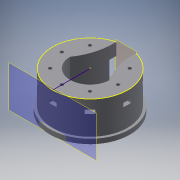
# Autodesk Inventor part: rotacion2_top
Saved by Autodesk Inventor 2017 (Build 210142000, 142)
## iProperties
Created: 2016-09-28
Part Number: rotacion2_top
Material: Generic
Document SubType Name: Modeling
Designer: Bardo91
Density: 1 g/cm^3
Appearance: Default
Author: Bardo91
Autodesk Inventor part; units mm, degrees
ref_plane "YZ Plane" through (0, 0, 0) normal (1, 0, 0) x (0, 1, 0)
ref_plane "XY Plane" through (0, 0, 0) normal (0, 0, 1) x (1, 0, 0)
sketch "Sketch1" plane through (0, 0, 0) normal (0, 0, 1) x (1, 0, 0)
  line L0 (0, -11) -> (-10.5, -11)
  line L1 (-10.5, -11) -> (-10.5, 31)
  line L2 (-10.5, 31) -> (10.5, 31)
  line L3 (10.5, 31) -> (10.5, -11)
  line L4 (10.5, -11) -> (0, -11)
  line L5 (10.5, 10) -> (0, 10)
  line L6 (0, 0) -> (0, 10)
  circle A0 centre (0, 0) radius 42.5
  dimension "d1" = 42
  dimension "d28" = 21
  dimension "d76" = 10
  dimension "d77" = 10.5
  dimension "d78" = 85
  constraints: 14 end point, 4 perpendicular, 2 horizontal, 1 centre point, 1 coincident, 1 midpoint, 1 point on line, 1 vertical, 1 other
  measures "d1" distance of L0.end L1.end
  measures "d28" distance of L1.end L2.end
  measures "d76" distance of L6.start L5.end
  measures "d77" distance of L0.start L0.end
  measures "d78" diameter of A0
extrude "Extrusion6" add sketch "Sketch1" along normal blind 5
sketch "Sketch9" plane through (0, 0, 5) normal (0, 0, 1) x (1, 0, 0)
  line L0 (10.5, -11) -> (-10.5, -11) projected
  line L1 (0, -11) -> (0, -14)
  line L2 (0, -14) -> (-5, -14)
  circle A0 centre (-5, -14) radius 3
  line L3 (0, -14) -> (5, -14)
  circle A1 centre (5, -14) radius 3
  line L4 (-10.5, -11) -> (-10.5, 31) projected
  line L5 (-10.5, 10) -> (10.5, 10)
  line L6 (10.5, 31) -> (-10.5, 31)
  line L7 (0, 31) -> (0, 34)
  line L8 (0, 34) -> (-5, 34)
  circle A2 centre (-5, 34) radius 3
  line L9 (0, 34) -> (5, 34)
  circle A3 centre (5, 34) radius 3
  dimension "d79" = 3
  dimension "d80" = 5
  dimension "d81" = 6
  dimension "d82" = 5
  dimension "d83" = 6
  constraints: 16 end point, 7 symmetric about line, 4 centre point, 4 coincident, 2 horizontal, 2 midpoint, 1 perpendicular, 1 vertical, 2 other
  measures "d79" distance of L1.start L1.end
  measures "d80" distance of L1.end L2.end
  measures "d81" diameter of A0
  measures "d82" distance of L1.end L3.end
  measures "d83" diameter of A1
extrude "Extrusion12" cut sketch "Sketch9" against normal through all contours A2 | A1 | A0 | A3
sketch "Sketch10" plane through (0, 0, 5) normal (0, 0, 1) x (1, 0, 0)
  line L0 (-10.5, 31) -> (-10.5, 38.5)
  circle A0 centre (0, 0) radius 39.9061
  line L1 (-10.5, -11) -> (-10.5, -18.5)
  arc A1 (-21.272, 0) -> (21.272, 0) centre (0, 0) ccw
  arc A2 (-21.272, 0) -> (-10.5, 31) centre (-71.284, 34.75) ccw
  line L2 (10.5, 31) -> (10.5, 38.5)
  arc A3 (10.5, 31) -> (21.272, 0) centre (71.284, 34.75) ccw
  dimension "d86" = 7.5
  dimension "d87" = 79.8123
  dimension "d88" = 7.5
  constraints: 11 point on circle, 6 end point, 4 centre point, 2 coincident, 2 point on line, 2 vertical
  measures "d86" distance of L0.start L0.end
  measures "d87" diameter of A0
  measures "d88" distance of L1.start L1.end
extrude "Extrusion13" add sketch "Sketch10" along normal blind 35 contours A2 A1 A3 L2 A0 L0 picked at (-28.5299, 15.6602)
sketch "Sketch11" plane through (0, 0, 40) normal (0, 0, 1) x (1, 0, 0)
  line L0 (0, 0) -> (0, -30)
  circle A0 centre (0, -30) radius 1.75
  circle A1 centre (21.2132, -21.2132) radius 1.75
  circle A2 centre (30, 0) radius 1.75
  circle A3 centre (21.2132, 21.2132) radius 1.75
  circle A4 centre (0, 30) radius 1.75
  circle A5 centre (-21.2132, 21.2132) radius 1.75
  circle A6 centre (-30, 0) radius 1.75
  circle A7 centre (-21.2132, -21.2132) radius 1.75
  dimension "d91" = 30
  dimension "d92" = 3.5
  dimension "d95" = 360
  constraints: 8 centre point, 3 coincident, 2 end point, 1 vertical, 23 other
  measures "d91" distance of L0.start L0.end
  measures "d92" diameter of A0
extrude "Extrusion14" cut sketch "Sketch11" against normal through all contours A0 | A1 | A2 | A3 | A5 | A6 | A7
sketch "Sketch12" plane through (0, 0, 40) normal (0, 0, 1) x (1, 0, 0)
  line L0 (0, 0) -> (0, -39.9061)
  arc A0 (-10.5, 38.5) -> (10.5, 38.5) centre (0, 0) ccw projected
  constraints: 2 end point, 1 point on circle, 1 vertical
ref_plane "Work Plane2" through (0, -39.9061, 40) normal (0, 1, 0) x (-1, 0, 0)
sketch "Sketch13" plane through (0, -39.9061, 40) normal (0, 1, 0) x (-1, 0, 0)
  line L0 (-0.0018, 0) -> (-0.0018, -10)
  line L1 (-0.0018, -10) -> (-4.0018, -10)
  line L2 (-4.0018, -10) -> (-4.0018, -14)
  line L3 (-4.0018, -14) -> (3.9982, -14)
  line L4 (3.9982, -14) -> (3.9982, -10)
  line L5 (3.9982, -10) -> (-0.0018, -10)
  point P0 (0, -40)
  dimension "d99" = 10
  dimension "d100" = 4
  dimension "d101" = 4
  dimension "d102" = 8
  constraints: 12 end point, 4 perpendicular, 2 vertical
  measures "d99" distance of L0.start L0.end
  measures "d100" distance of L0.end L1.end
  measures "d101" distance of L1.end L2.end
  measures "d102" distance of L2.end L3.end
extrude "Extrusion15" cut sketch "Sketch13" along normal blind 15
pattern_circular "Circular Pattern2" count 8 over 360 about axis through (0, 0, 5) along (0, 0, 1) of "Extrusion15"
ref_plane "Work Plane3" through (10.5, 38.5, 40) normal (0, -1, 0) x (-1, 0, 0)
sketch "Sketch14" plane through (10.5, 38.5, 40) normal (0, -1, 0) x (-1, 0, 0)
  line L0 (0, 35) -> (5.5, 35) projected
  line L1 (-10.772, 35) -> (-10.772, 0) projected
  line L2 (-10, 35) -> (-8, 35) construction
  line L3 (-10, 33) -> (0, 33)
  line L4 (-10, 33) -> (-10, 13)
  line L5 (-9.941, 10) -> (-9.941, 14) projected
  line L6 (-10, 33) -> (10, 33) construction
  line L7 (-10, 13) -> (0, 13)
  line L8 (0, 13) -> (0, 33)
  line L9 (0, 35) -> (0, 0) projected
  line L10 (21, 35) -> (21, 0) projected
  line L11 (21, 33) -> (31, 33)
  line L12 (31, 33) -> (31, 13)
  line L13 (31, 13) -> (21, 13)
  line L14 (21, 13) -> (21, 33)
  point P0 (10.5, 40)
  dimension "d109" = 2
  dimension "d111" = 20
  dimension "d112" = 90
  dimension "d113" = 10
  dimension "d114" = 20
  constraints: 20 end point, 5 perpendicular, 2 horizontal, 1 collinear, 1 parallel, 1 point on line
  measures "d109" distance of L2.start L3.start
  measures "d111" distance of L3.start L4.end
  measures "d112" angle of L4 L6
  measures "d113" distance of L11.start L11.end
  measures "d114" distance of L11.end L12.end
extrude "Extrusion16" cut sketch "Sketch14" along normal blind 7.5
sketch "Sketch15" plane through (10.5, 31, 40) normal (0, 1, 0) x (1, 0, 0)
  line L0 (-21, 13) -> (-21, 0) projected
  line L1 (-31, 13) -> (-31, 33) projected
  line L2 (-21, 33) -> (-21, 13) projected
  line L3 (0, 35) -> (0, 33) projected
  line L4 (10, 13) -> (0, 13) projected
  line L5 (0, 33) -> (10, 33) projected
  circle A0 centre (5, 23) radius 1.5
  circle A1 centre (-26, 23) radius 1.5
  point P0 (-10.5, 40)
  dimension "d118" = 3
  dimension "d119" = 3
  constraints: 2 centre point
  measures "d118" diameter of A0
  measures "d119" diameter of A1
extrude "Extrusion17" cut sketch "Sketch15" against normal blind 5
body "Solid2"
